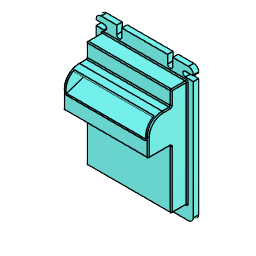
TB74 (Autodesk Fusion 360 design; units mm, degrees)
Autodesk Fusion 360 part; units mm, degrees
sketch "Sketch1" plane through (0, 0, 0) normal (0, 1, 0) x (1, 0, 0) in component "TB74"
  line L0 (-48.75, -67) -> (48.75, -67)
  line L1 (48.75, -67) -> (48.75, 67)
  line L2 (48.75, 67) -> (-48.75, 67)
  line L3 (-48.75, 67) -> (-48.75, -67)
  line L4 (-48.75, -67) -> (48.75, 67) construction
  line L5 (48.75, -67) -> (-48.75, 67) construction
  dimension "d1" = 97.5
  dimension "d2" = 134
  constraint horizontal L0
  constraint perpendicular L0 L1
  constraint parallel L0 L2
  constraint parallel L1 L3
  constraint coincident L4 origin
  constraint coincident L5 origin
  measures "d1" distance of L1.end L2.end
  measures "d2" distance of L0.end L1.end
extrude "Extrude1" add sketch "Sketch1" against normal blind 5.5 in component "TB74"
sketch "Sketch2" plane through (0, -5.5, 0) normal (0, -1, 0) x (1, 0, 0) in component "TB74"
  line L0 (-48.75, 67) -> (-48.75, -67)
  line L1 (-48.75, -67) -> (48.75, -67)
  line L2 (48.75, -67) -> (48.75, 67)
  line L3 (48.75, 67) -> (-48.75, 67)
  line L4 (-42.5, 53.75) -> (42.5, 53.75)
  line L5 (42.5, 53.75) -> (42.5, -53.75)
  line L6 (42.5, -53.75) -> (-42.5, -53.75)
  line L7 (-42.5, -53.75) -> (-42.5, 53.75)
  line L8 (-42.5, 53.75) -> (42.5, -53.75) construction
  line L9 (42.5, 53.75) -> (-42.5, -53.75) construction
  dimension "d5" = 85
  dimension "d6" = 107.5
  constraint horizontal L4
  constraint perpendicular L4 L5
  constraint parallel L4 L6
  constraint parallel L5 L7
  constraint coincident L8 origin
  constraint coincident L9 origin
  measures "d5" distance of L5.end L6.end
  measures "d6" distance of L4.end L5.end
extrude "Extrude2" add sketch "Sketch2" along normal blind 16 contours L4 L5 L6 L7 in component "TB74"
sketch "Sketch3" plane through (0, -21.5, 0) normal (0, -1, 0) x (1, 0, 0) in component "TB74"
  line L0 (-42.5, -53.75) -> (42.5, -53.75)
  line L1 (42.5, -53.75) -> (42.5, 53.75)
  line L2 (42.5, 53.75) -> (-42.5, 53.75)
  line L3 (-42.5, 53.75) -> (-42.5, -53.75)
  line L4 (0, 53.75) -> (0, 39) construction
  line L5 (0, 39) -> (42.5, 39)
  line L6 (0, 39) -> (-42.5, 39)
  line L7 (-42.5, 39) -> (-42.5, 5.5)
  line L8 (-42.5, 5.5) -> (42.5, 5.5)
  line L9 (42.5, 5.5) -> (42.5, 39)
  dimension "d9" = 14.75
  dimension "d10" = 33.5
  constraint midpoint L2 L4.start
  constraint perpendicular L2 L4
  constraint coincident L1 L5.end
  constraint perpendicular L1 L5
  constraint coincident L3 L6.end
  constraint perpendicular L3 L6
  constraint perpendicular L6 L7
  constraint coincident L1 L8.end
  constraint perpendicular L1 L8
  measures "d9" distance of L4.start L4.end
  measures "d10" distance of L6.end L7.end
extrude "Extrude3" add sketch "Sketch3" along normal blind 23 contours L1 L3 L5 L6 L7 L8 L9 in component "TB74"
sketch "Sketch4" plane through (0, -44.5, 0) normal (0, -1, 0) x (1, 0, 0) in component "TB74"
  line L0 (42.5, 39) -> (-42.5, 39)
  line L1 (-42.5, 39) -> (-42.5, 5.5)
  line L2 (-42.5, 5.5) -> (42.5, 5.5)
  line L3 (42.5, 5.5) -> (42.5, 39)
  line L4 (0, 39) -> (0, 5.5) construction
  line L5 (-40, 35.5727) -> (40, 35.5727)
  line L6 (40, 35.5727) -> (40, 30.5727)
  line L7 (40, 30.5727) -> (-40, 30.5727)
  line L8 (-40, 30.5727) -> (-40, 35.5727)
  line L9 (-40, 35.5727) -> (40, 30.5727) construction
  line L10 (40, 35.5727) -> (-40, 30.5727) construction
  point P0 (0, 33.0727)
  dimension "d13" = 80
  dimension "d14" = 5
  constraint midpoint L0 L4.start
  constraint midpoint L2 L4.end
  constraint horizontal L5
  constraint perpendicular L5 L6
  constraint parallel L5 L7
  constraint parallel L6 L8
  constraint coincident L9 P0
  constraint coincident L10 P0
  constraint coincident L4 P0
  measures "d13" distance of L6.end L7.end
  measures "d14" distance of L5.end L6.end
extrude "Extrude4" cut sketch "Sketch4" against normal blind 44.5 contours L5 L6 L7 L8 in component "TB74"
chamfer "Chamfer1" distance 10 distance2 30 1 edges at (0, -44.5, 30.5727) measured on face at (-13.3333, -44.5, 13.8576) in component "TB74"
fillet "Fillet1" radius 15 1 edges at (0, -44.5, 39) in component "TB74"
fillet "Fillet2" radius 5 4 edges at (48.75, -2.75, 67) (-48.75, -2.75, 67) (-48.75, -2.75, -67) (48.75, -2.75, -67) in component "TB74"
fillet "Fillet3" radius 1 27 edges at (42.5, -44.5, 14.75) (42.5, -40.1066, 34.6066) (42.5, -25.5, 39) (-42.5, -25.5, 39) (-42.5, -40.1066, 34.6066) (-42.5, -44.5, 14.75) (0, -21.5, 39) (0, -21.5, 53.75) (42.5, -21.5, 46.375) (42.5, -13.5, 53.75) (0, -5.5, 53.75) (42.5, -5.5, 0) (-42.5, -21.5, 46.375) (-42.5, -13.5, 53.75) (-42.5, -5.5, 0) (-42.5, -33, 5.5) (0, -44.5, 5.5) (0, -44.5, 20.5727) (0, -39.0432, 35.5727) (-42.5, -21.5, -24.125) (42.5, -21.5, -24.125) (42.5, -33, 5.5) (0, -21.5, 5.5) (0, -21.5, -53.75) (42.5, -13.5, -53.75) (0, -5.5, -53.75) (-42.5, -13.5, -53.75) in component "TB74"
sketch "Sketch5" plane through (0, -5.5, 0) normal (0, -1, 0) x (1, 0, 0) in component "TB74"
  arc A0 (43.75, -67) -> (48.75, -62) centre (43.75, -62) ccw
  line L0 (48.75, -62) -> (48.75, 62)
  arc A1 (48.75, 62) -> (43.75, 67) centre (43.75, 62) ccw
  line L1 (43.75, 67) -> (-43.75, 67)
  arc A2 (-43.75, 67) -> (-48.75, 62) centre (-43.75, 62) ccw
  line L2 (-48.75, 62) -> (-48.75, -62)
  arc A3 (-48.75, -62) -> (-43.75, -67) centre (-43.75, -62) ccw
  line L3 (-43.75, -67) -> (43.75, -67)
  arc A4 (43.5, 52.75) -> (41.5, 54.75) centre (41.5, 52.75) ccw
  line L4 (43.5, 52.75) -> (43.5, -52.75)
  arc A5 (41.5, -54.75) -> (43.5, -52.75) centre (41.5, -52.75) ccw
  line L5 (41.5, -54.75) -> (-41.5, -54.75)
  arc A6 (-43.5, -52.75) -> (-41.5, -54.75) centre (-41.5, -52.75) ccw
  line L6 (-43.5, -52.75) -> (-43.5, 52.75)
  arc A7 (-41.5, 54.75) -> (-43.5, 52.75) centre (-41.5, 52.75) ccw
  line L7 (-41.5, 54.75) -> (41.5, 54.75)
  line L8 (0, 67) -> (0, 54.75) construction
  line L9 (-25.5, 63.0222) -> (25.5, 63.0222) construction
  line L10 (25.5, 63.0222) -> (25.5, 58.7278) construction
  line L11 (25.5, 58.7278) -> (-25.5, 58.7278) construction
  line L12 (-25.5, 58.7278) -> (-25.5, 63.0222) construction
  line L13 (-25.5, 63.0222) -> (25.5, 58.7278) construction
  line L14 (25.5, 63.0222) -> (-25.5, 58.7278) construction
  circle A8 centre (-25.5, 58.7278) radius 2.5
  circle A9 centre (25.5, 58.7278) radius 2.5
  line L15 (-25.5, 58.7278) -> (25.5, 58.7278) construction
  line L16 (-25.5, 58.7278) -> (-28, 58.7278) construction
  line L17 (25.5, 58.7278) -> (28, 58.7278) construction
  line L18 (-28, 58.7278) -> (-28, 67)
  line L19 (-23, 58.7278) -> (-23, 67)
  line L20 (23, 58.7278) -> (23, 67)
  line L21 (28, 58.7278) -> (28, 67)
  line L22 (-25.5, 58.7278) -> (-48.75, 58.7278) construction
  line L23 (28, 58.7278) -> (48.75, 58.7278) construction
  line L24 (-48.75, 58.7278) -> (-40.75, 58.7278) construction
  line L25 (48.75, 58.7278) -> (40.75, 58.7278) construction
  circle A10 centre (-40.75, 58.7278) radius 2.5
  circle A11 centre (40.75, 58.7278) radius 2.5
  line L26 (-40.75, 58.7278) -> (-40.75, 67) construction
  line L27 (-40.75, 58.7278) -> (-40.75, 54.75) construction
  line L28 (40.75, 58.7278) -> (40.75, 67) construction
  line L29 (40.75, 58.7278) -> (40.75, 54.75) construction
  line L30 (-40.75, 61.2278) -> (-48.75, 61.2278)
  line L31 (-40.75, 56.2278) -> (-48.75, 56.2278)
  line L32 (40.75, 61.2278) -> (48.75, 61.2278)
  line L33 (40.75, 56.2278) -> (48.75, 56.2278)
  point P0 (0, 60.875)
  dimension "d25" = 51
  dimension "d26" = 5
  dimension "d27" = 5
  dimension "d30" = 8
  dimension "d31" = 8
  dimension "d32" = 5
  dimension "d33" = 5
  constraint midpoint L1 L8.start
  constraint midpoint L7 L8.end
  constraint horizontal L9
  constraint perpendicular L9 L10
  constraint parallel L9 L11
  constraint parallel L10 L12
  constraint coincident L13 P0
  constraint coincident L14 P0
  constraint midpoint L8 P0
  constraint coincident L11.end L12.start
  constraint coincident L10.end L11.start
  constraint coincident A8 L16.end
  constraint perpendicular L12 L16
  constraint coincident A9 L17.end
  constraint parallel L15 L17
  constraint coincident L1 L18.end
  constraint perpendicular L1 L18
  constraint coincident L11 L19.start
  constraint coincident A8 L19.start
  constraint coincident L1 L19.end
  constraint tangent A8 L19
  constraint coincident A9 L20.start
  constraint coincident L15 L20.start
  constraint coincident L1 L20.end
  constraint tangent A9 L20
  constraint coincident L1 L21.end
  constraint perpendicular L1 L21
  constraint coincident L2 L22.end
  constraint perpendicular L2 L22
  constraint coincident L0 L23.end
  constraint perpendicular L0 L23
  constraint perpendicular L2 L24
  constraint perpendicular L0 L25
  constraint coincident L24.end A10.centre
  constraint coincident L25.end A11.centre
  constraint coincident L1 L26.end
  constraint perpendicular L1 L26
  constraint coincident L7 L27.end
  constraint perpendicular L7 L27
  constraint coincident L1 L28.end
  constraint perpendicular L1 L28
  constraint coincident L7 L29.end
  constraint perpendicular L7 L29
  constraint coincident A10 L30.start
  constraint coincident L26 L30.start
  constraint coincident L2 L30.end
  constraint tangent A10 L30
  constraint coincident A10 L31.start
  constraint coincident L27 L31.start
  constraint coincident L2 L31.end
  constraint tangent A10 L31
  constraint coincident L28 L32.start
  constraint coincident A11 L32.start
  constraint coincident L0 L32.end
  constraint tangent A11 L32
  constraint coincident A11 L33.start
  constraint coincident L29 L33.start
  constraint coincident L0 L33.end
  constraint tangent A11 L33
  measures "d25" distance of L10.end L11.end
  measures "d26" diameter of A8
  measures "d27" diameter of A9
  measures "d30" distance of L22.end L24.end
  measures "d31" distance of L23.end L25.end
  measures "d32" diameter of A10
  measures "d33" diameter of A11
extrude "Extrude5" cut sketch "Sketch5" against normal blind 6 contours L0 A11 L32 L33 | A11 | L2 A10 L30 L31 | A10 | L1 A9 L20 L21 | A9 | L1 A8 L18 L19 | A8 in component "TB74"
component "TB74" placed x (1, 0, 0) y (0, 1, 0) z (0, 0, 1) at (0, 0, 0)
